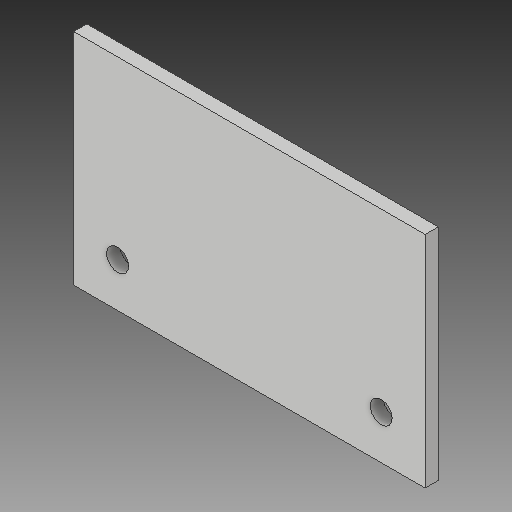
# Autodesk Inventor part: 車軸受け板
Saved by Autodesk Inventor 2017 (Build 210142000, 142)
## iProperties
Part Number: 車軸受け板
Material: 一般
Document SubType Name: Modeling
Designer: highs
Density: 1 g/cm^3
Appearance: 既定
Author: highs
Autodesk Inventor part; units mm, degrees
ref_plane "YZ Plane" through (0, 0, 0) normal (1, 0, 0) x (0, 1, 0)
ref_plane "XZ Plane" through (0, 0, 0) normal (0, 1, 0) x (-1, 0, 0)
ref_plane "XY Plane" through (0, 0, 0) normal (0, 0, 1) x (1, 0, 0)
sketch "スケッチ1" plane through (0, 0, 0) normal (0, 0, 1) x (1, 0, 0)
  line L0 (0, 0) -> (80, 0)
  line L1 (80, 0) -> (80, 50)
  line L2 (40, 0) -> (40, 73.3333) construction
  line L3 (0, 50) -> (0, 0)
  circle A0 centre (10, 10) radius 2.5
  circle A1 centre (70, 10) radius 2.5
  line L4 (10, 10) -> (70, 10) construction
  line L5 (0, 50) -> (80, 50)
  dimension "d2" = 80
  dimension "d6" = 5
  dimension "d7" = 10
  dimension "d14" = 10
  dimension "d17" = 50
  constraints: 12 end point, 3 horizontal, 2 centre point, 1 midpoint, 1 parallel, 1 perpendicular, 1 symmetric about line, 1 vertical, 2 other
  measures "d2" distance of L0.start L0.end
  measures "d6" diameter of A0
  measures "d7" distance from line of L3 L4.start
  measures "d14" distance between parallel lines of L0 L4
  measures "d17" distance of L3.start L0.start
extrude "押し出し1" add sketch "スケッチ1" along normal blind 3
